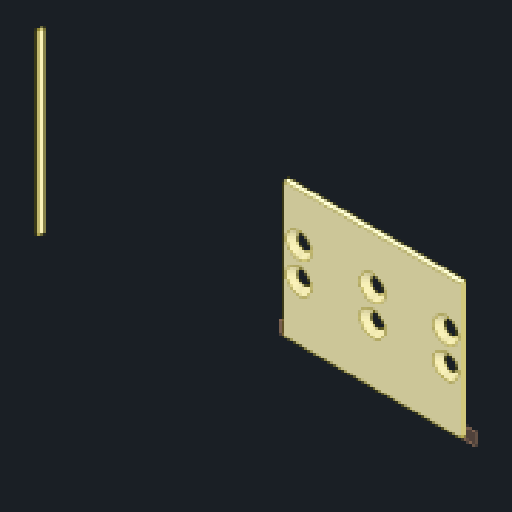
# Autodesk Inventor part: back
Saved by Autodesk Inventor 2023 (Build 270158000, 158)
## iProperties
Created: 2024-04-24
Part Number: back
Material: Nylon 6/6
Document SubType Name: Modeling
Designer: szymo
Density: 1.13 g/cm^3
Appearance: Nylon 6
Mass: 13.0286 g
Surface Area: 172.827 cm^2
Volume: 11.5297 cm^3
Author: szymo
Autodesk Inventor part; units mm, degrees
ref_plane "YZ Plane" through (0, 0, 0) normal (1, 0, 0) x (0, 1, 0)
ref_plane "XZ Plane" through (0, 0, 0) normal (0, 1, 0) x (-1, 0, 0)
ref_plane "XY Plane" through (0, 0, 0) normal (0, 0, 1) x (1, 0, 0)
ref_plane "Work Plane1" through (0, 0, 0) normal (0, 0, 1) x (1, 0, 0)
sketch "Sketch1" plane through (0, 0, 0) normal (0, 0, 1) x (1, 0, 0)
  line L0 (47, 1) -> (47, 3) projected
  line L1 (0, 3) -> (47, 3) projected
  line L2 (0, 1) -> (0, 3) projected
  line L3 (-65.5, 38.5) -> (112.5, 38.5)
  line L4 (112.5, 38.5) -> (112.5, -8.5)
  line L5 (112.5, -8.5) -> (-65.5, -8.5)
  line L6 (-65.5, -8.5) -> (-65.5, 38.5)
  line L7 (-65, -11.5) -> (-65, 38.5) projected
  line L8 (0, 1) -> (47, 1) projected
  line L9 (46, 36.5) -> (46, 3) projected
  line L10 (46, 3) -> (47, 3) projected
  line L11 (47, 36.5) -> (47, 3) projected
  line L12 (46, 36.5) -> (47, 36.5) projected
  line L13 (1, 36.5) -> (1, 3) projected
  line L14 (1, 36.5) -> (0, 36.5) projected
  line L15 (0, 36.5) -> (0, 3) projected
  line L16 (1, 3) -> (0, 3) projected
  line L17 (0, 36.5) -> (47, 36.5)
  line L18 (47, 36.5) -> (47, 1)
  line L19 (47, 1) -> (0, 1)
  line L20 (0, 1) -> (0, 36.5)
  point P0 (23.5, 0)
  point P1 (-65, -8.5)
  dimension "d0" = 178
  dimension "d1" = 89
  dimension "d2" = 89
  dimension "d3" = 0
  dimension "d13" = 3
  constraints: 16 end point, 4 parallel, 2 horizontal, 2 perpendicular
  measures "d0" distance of L3.start L3.end
  measures "d1" distance from line of L6 point (23.5, 0)
  measures "d2" distance from line of L4 point (23.5, 0)
  measures "d3" distance from line of L3 L7.end
  measures "d13" distance from line of L5 L7.start
extrude "Extrusion1" add sketch "Sketch1" along normal blind 1.4 contours L8 L2 L1 L0 | L1 L9 L12 L11 | L1 L13 L17 L9 | L15 L14 L13 L1
sketch "Sketch2" plane through (0, 0, 1.4) normal (0, 0, 1) x (1, 0, 0)
  circle A0 centre (4, 23.825) radius 2.3 projected
  circle A1 centre (4, 15.675) radius 2.3 projected
  line L0 (7, 36.5) -> (1, 36.5) projected
  line L1 (1, 3) -> (1, 36.5) projected
  line L2 (1, 3) -> (7, 3) projected
  line L3 (7, 3) -> (7, 36.5) projected
  circle A2 centre (23.5, 23.825) radius 2.3 projected
  circle A3 centre (23.5, 15.675) radius 2.3 projected
  line L4 (28, 36.5) -> (19, 36.5) projected
  line L5 (19, 3) -> (19, 36.5) projected
  line L6 (19, 3) -> (28, 3) projected
  line L7 (28, 3) -> (28, 36.5) projected
  circle A4 centre (43, 23.825) radius 2.3 projected
  circle A5 centre (43, 15.675) radius 2.3 projected
  line L8 (46, 36.5) -> (40, 36.5) projected
  line L9 (40, 3) -> (40, 36.5) projected
  line L10 (40, 3) -> (46, 3) projected
  line L11 (46, 3) -> (46, 36.5) projected
  point P0 (0, 0)
  constraints: 6 coincident
hole "Hole1" at (4, 23.825, 1.4) at (4, 15.675, 1.4) at (23.5, 15.675, 1.4) at (23.5, 23.825, 1.4) at (43, 23.825, 1.4) at (43, 15.675, 1.4) direction (0, 0, -1) diameter 3.6 end through all countersink diameter 6.6 countersink angle 90 clearance for "Countersunk Flat Head Screw ISO 2009/7046" size "M3" standard "ISO"
equation "\"d1\" = d2"
body "Solid1"
